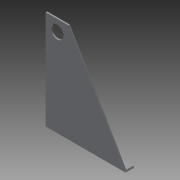
# Autodesk Inventor part: RPlate
Saved by Autodesk Inventor 2013 (Build 170138000, 138)
## iProperties
Created: 2014-01-21
Part Number: RPlate
Material: Generic
Document SubType Name: Modeling
Designer: RobertB
Density: 1 g/cm^3
Author: RobertB
Autodesk Inventor part; units mm, degrees
ref_plane "YZ Plane" through (0, 0, 0) normal (1, 0, 0) x (0, 1, 0)
ref_plane "XZ Plane" through (0, 0, 0) normal (0, 1, 0) x (-1, 0, 0)
ref_plane "XY Plane" through (0, 0, 0) normal (0, 0, 1) x (1, 0, 0)
sketch "Sketch1" plane through (0, 0, 0) normal (0, 0, 1) x (1, 0, 0)
  line L0 (25.4, -110.3376) -> (-25.4, -110.3376)
  line L1 (-25.4, -110.3376) -> (-25.4, 110.3376)
  line L2 (-25.4, 110.3376) -> (25.4, 110.3376)
  line L3 (25.4, 110.3376) -> (25.4, -110.3376)
  line L4 (25.4, -110.3376) -> (-25.4, 110.3376) construction
  line L5 (-25.4, -110.3376) -> (25.4, 110.3376) construction
  line L6 (25.4, 110.3376) -> (152.8069, -110.3376)
  line L7 (25.4, 110.3376) -> (280.2138, 110.3376) construction
  line L8 (152.8069, -110.3376) -> (25.4, -110.3376)
  point P0 (0, 0)
  dimension "d0" = 50.8
  dimension "d1" = 220.6752
  dimension "d2" = 60
  constraints: 18 end point, 2 horizontal, 2 midpoint, 2 parallel, 1 collinear, 1 equal length, 1 perpendicular
  measures "d0" distance of L1.end L2.end
  measures "d1" distance of L0.end L1.end
  measures "d2" angle of L6 L7
extrude "Extrusion1" add sketch "Sketch1" along normal blind 3.175
sketch "Sketch2" plane through (0, 0, 3.175) normal (0, 0, 1) x (1, 0, 0)
  line L0 (152.8069, -110.3376) -> (25.4, 110.3376) projected
  line L1 (-25.4, -110.3376) -> (152.8069, -110.3376)
  line L2 (152.8069, -107.1626) -> (-25.4, -107.1626)
  line L3 (-25.4, -107.1626) -> (-25.4, -110.3376)
  line L4 (150.9738, -107.1626) -> (152.8069, -110.3376)
  point P0 (0, 0)
  dimension "d5" = 3.175
  constraints: 8 end point, 2 point on line, 1 collinear, 1 horizontal, 1 parallel
  measures "d5" distance of L2.start L1.end
extrude "Extrusion2" add sketch "Sketch2" against normal blind 19.05
sketch "Sketch3" plane through (0, 0, 3.175) normal (0, 0, 1) x (1, 0, 0)
  line L0 (-25.4, 110.3376) -> (0, 110.3376)
  line L1 (0, 110.3376) -> (0, 84.9376)
  line L2 (0, 84.9376) -> (-25.4, 84.9376)
  line L3 (-25.4, 84.9376) -> (-25.4, 110.3376)
  circle A0 centre (0, 84.9376) radius 14.2875
  point P0 (0, 0)
  dimension "d8" = 25.4
  dimension "d9" = 25.4
  dimension "d10" = 28.575
  constraints: 8 end point, 2 parallel, 1 centre point, 1 coincident, 1 horizontal, 1 perpendicular
  measures "d8" distance of L1.end L2.end
  measures "d9" distance of L0.end L1.end
  measures "d10" diameter of A0
extrude "Extrusion3" cut sketch "Sketch3" against normal blind 25.4 contours A0 L2 L1 | L1 L2 A0
body "Solid1"
